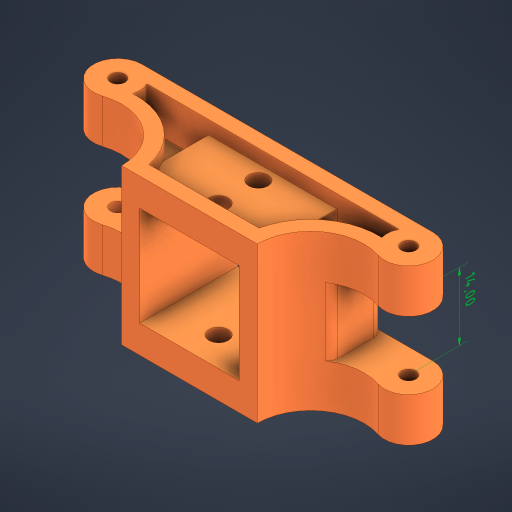
# Autodesk Inventor part: shock_absorber_holder_up
Saved by Autodesk Inventor 2024 (Build 280153000, 153)
## iProperties
Created: 2023-05-07
Part Number: shock_absorber_holder_up
Material: Типовые
Document SubType Name: Modeling
Designer: user
Density: 1 g/cm^3
Appearance: По умолчанию
Author: user
Autodesk Inventor part; units mm, degrees
ref_plane "YZ Plane" through (0, 0, 0) normal (1, 0, 0) x (0, 1, 0)
ref_plane "XZ Plane" through (0, 0, 0) normal (0, 1, 0) x (-1, 0, 0)
sketch "Эскиз1" plane through (0, 0, 0) normal (0, 0, 1) x (1, 0, 0)
  line L0 (0, 0) -> (14, 0)
  arc A0 (28.4375, 10.4491) -> (14, 0) centre (25, 0) ccw
  arc A1 (28.4375, 10.4491) -> (30, 20.1987) centre (30, 15.1987) ccw
  line L1 (30, 20.1987) -> (-30, 20.1987)
  arc A2 (-30, 20.1987) -> (-28.4375, 10.4491) centre (-30, 15.1987) ccw
  line L2 (0, 0) -> (-14, 0)
  arc A3 (-14, 0) -> (-28.4375, 10.4491) centre (-25, 0) ccw
  circle A4 centre (-30, 15.1987) radius 1.5
  circle A5 centre (30, 15.1987) radius 1.5
  point P0 (0, 20.1987)
  dimension "d2" = 3
  dimension "d5" = 28
  dimension "d6" = 11
  dimension "d7" = 5
  dimension "d8" = 60
  constraints: 8 point on circle, 6 centre point, 6 end point, 4 tangent, 3 horizontal, 2 coincident, 2 line through centre, 1 collinear, 1 equal radius, 1 horizontal alignment, 1 midpoint, 1 vertical alignment
  measures "d2" diameter of A5
  measures "d5" distance of L0.end L2.end
  measures "d6" radius of A0
  measures "d7" radius of A1
  measures "d8" distance of L1.start L1.end
extrude "Выдавливание1" add sketch "Эскиз1" along normal blind 28
sketch "Эскиз2" plane through (-14, 0, 0) normal (0, -1, 0) x (1, 0, 0)
  line L0 (3.75, 3.75) -> (24.25, 3.75)
  line L1 (24.25, 3.75) -> (24.25, 24.25)
  line L2 (24.25, 24.25) -> (3.75, 24.25)
  line L3 (3.75, 24.25) -> (3.75, 3.75)
  line L4 (0, 28) -> (28, 28) projected
  line L5 (28, 0) -> (28, 28) projected
  point P0 (14, 0)
  point P1 (14, 24.25)
  point P2 (14, 28)
  point P3 (24.25, 14)
  point P4 (28, 14)
  dimension "d11" = 20.5
  constraints: 8 end point, 4 midpoint, 2 parallel, 2 perpendicular, 1 horizontal, 1 horizontal alignment, 1 vertical alignment
  measures "d11" distance of L1.end L2.end
extrude "Выдавливание2" cut sketch "Эскиз2" against normal blind 28
ref_plane "РабПлоскость2" through (35, 15.1987, 0) normal (1, 0, 0) x (0, 0, -1)
ref_plane "РабПлоскость1" through (0, 20.1987, 28) normal (1, 0, 0) x (0, 0, -1)
sketch "Эскиз4" plane through (35, 15.1987, 0) normal (1, 0, 0) x (0, 0, -1)
  line L0 (0, 5) -> (-28, 5) projected
  line L1 (0, -5) -> (-28, -5) projected
  line L2 (-19, 5) -> (-9, 5)
  line L3 (-9, 5) -> (-9, -5)
  line L4 (-9, -5) -> (-19, -5)
  line L5 (-19, -5) -> (-19, 5)
  point P0 (0, -15.1987)
  point P1 (-14, -5)
  point P2 (-14, -5)
  point P3 (-19, -5)
  dimension "d24" = 10
  constraints: 8 end point, 2 midpoint, 2 parallel, 2 point on line, 1 coincident, 1 horizontal, 1 perpendicular
  measures "d24" distance of L4.end L3.end
extrude "Выдавливание4" cut sketch "Эскиз4" against normal blind 15.25
mirror "Зеркальное отражение1" about plane through (0, 20.1987, 28) normal (1, 0, 0) of "Выдавливание4"
move faces "Перенос3" translate (0, -7, 0) faces at (20.5023, 10.1987, 15.6667)
move faces "Перенос4" translate (0, -8, 0) faces at (-20.5023, 10.1987, 15.6667)
shell "Оболочка3" thickness 3 removed faces 2 at (-6.1836, 16.4361, 0) at (-6.1836, 16.4361, 28)
sketch "Эскиз5" plane through (-13.25, 17.1987, 27.25) normal (0, 0, 1) x (1, 0, 0)
  circle A0 centre (13.25, -3) radius 2
  circle A1 centre (13.25, -11.1987) radius 2
  line L0 (43.25, 3) -> (-16.75, 3) projected
  line L1 (-0.75, -17.1987) -> (27.25, -17.1987) projected
  point P0 (13.25, -17.1987)
  point P1 (13.25, 3)
  point P2 (13.25, -17.1987)
  point P3 (13.25, -17.1987)
  point P4 (13.25, 3)
  dimension "d35" = 6
  dimension "d36" = 6
  dimension "d37" = 4
  constraints: 4 midpoint, 2 centre point, 2 vertical alignment, 1 equal radius
  measures "d35" distance of A1.centre point (13.25, -17.199)
  measures "d36" distance of point (13.25, 3) A0.centre
  measures "d37" diameter of A0
extrude "Выдавливание5" cut sketch "Эскиз5" against normal blind 31.75
fillet "Сопряжение1" radius 2 4 edges at (19.75, 20.1987, 14) (-19.75, 20.1987, 14) (19.75, 9.6663, 14) (-19.75, 9.6663, 14)
move faces "Перенос5" translate (0, 0, 2) faces at (8.6563, 19.1987, 28)
move faces "Перенос6" translate (0, 0, -2) faces at (-8.6563, 19.1987, 0)
move faces "Перенос7" translate (0, 0, 2) faces at (23.9163, 14.7648, 19)
move faces "Перенос8" translate (0, 0, -2) faces at (23.9163, 14.7648, 9)
move faces "Перенос9" translate (0, 0, 2) faces at (-23.9163, 14.7648, 19)
move faces "Перенос10" translate (0, 0, -2) faces at (-23.9163, 14.7648, 9)
equation "\"d36\" = d35"
